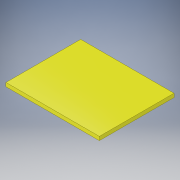
# Autodesk Inventor part: LargeCaseCaseTopForPiZeroWV02
Saved by Autodesk Inventor 2019.4 (Build 234330000, 330)
## iProperties
Created: 2018-12-18
Part Number: LargeCaseCaseTopForPiZeroWV02
Material: LCP Plastic
Document SubType Name: Modeling
Designer: steele
Density: 1.626 g/cm^3
Appearance: Yellow
PiZeroWLength: 2.559 in
PiZeroWWidth: 1.181 in
CaseLength: 3.150 in
CaseWidth: 1.772 in
CaseHeight: 0.515 in
PiZeroWMountingHole: 0.108 in
CaseWallThickness: 0.050 in
CaseFloorThickness: 0.200 in
PiZeroMoutingHolesLength: 2.283 in
PiZeroMountingHolesWidth: 0.906 in
PiZeroHoleSupport: 0.236 in
PiZeroWHoleHeight: 0.100 in
PiRibbonCableWidth: 0.787 in
PiRibbonCableThickness: 0.197 in
HdmiCenter: 0.748 in
MiniUsbCenter: 1.630 in
PowerCenter: 2.126 in
HdmiWidth: 1.102 in
MiniUsbWidth: 0.709 in
PowerWidth: 0.787 in
EndOfCaseToStartOfPiZero: 0.295 in
EyepieceOutsideDiameter: 1.250 in
EyepieceWallThickness: 0.075 in
EyepieceInnerDiameter: 1.100 in
PiRibbonCableHeightFromTp: 0.350 in
NutHeightPlusOffset: 0.073 in
NutWidthPlusOffset: 0.198 in
Author: steele
Autodesk Inventor part; units mm, degrees
ref_plane "YZ Plane" through (0, 0, 0) normal (1, 0, 0) x (0, 1, 0)
ref_plane "XZ Plane" through (0, 0, 0) normal (0, 1, 0) x (-1, 0, 0)
ref_plane "XY Plane" through (0, 0, 0) normal (0, 0, 1) x (1, 0, 0)
sketch "Sketch1" plane through (0, 0, 0) normal (0, 1, 0) x (-1, 0, 0)
  line L0 (63.5, 50.8) -> (-63.5, 50.8)
  line L1 (-63.5, 50.8) -> (-63.5, -50.8)
  line L2 (-63.5, -50.8) -> (63.5, -50.8)
  line L3 (63.5, -50.8) -> (63.5, 50.8)
  line L4 (63.5, 50.8) -> (-63.5, -50.8) construction
  line L5 (-63.5, 50.8) -> (63.5, -50.8) construction
  point P0 (0, 0)
  dimension "d0" = 127
  dimension "d1" = 101.6
  constraints: 12 end point, 2 midpoint, 2 parallel, 1 horizontal, 1 perpendicular
  measures "d0" distance of L1.end L2.end
  measures "d1" distance of L2.end L0.start
extrude "Extrusion1" add sketch "Sketch1" against normal blind 5.08
sketch "Sketch22" plane through (0, -5.08, 0) normal (0, -1, 0) x (1, 0, 0)
  point P0 (34.92, -17.42)
  point P1 (34.92, 17.42)
  point P2 (-34.92, 17.42)
  point P3 (-34.92, -17.42)
equation "\"d0\" = LargeCaseLength"
equation "\"d1\" = LargeCaseWidth"
equation "\"d2\" = CaseFloorThickness"
equation "\"PiZeroWLength\" = 65"
equation "\"PiZeroWWidth\" = 30"
equation "\"CaseLength\" = PiZeroWLength + 2 * EndOfCaseToStartOfPiZero"
equation "\"CaseWidth\" = PiZeroWWidth + 2 * EndOfCaseToStartOfPiZero"
equation "\"PiZeroWMountingHole\" = 2.75"
equation "\"CaseWallThickness\" = 1.27"
equation "\"CaseFloorThickness\" = 5.08"
equation "\"PiZeroMoutingHolesLength\" = 58"
equation "\"PiZeroMountingHolesWidth\" = 23"
equation "\"PiZeroHoleSupport\" = 6"
equation "\"PiZeroWHoleHeight\" = 2.54"
equation "\"PiRibbonCableWidth\" = 20"
equation "\"PiRibbonCableThickness\" = 5"
equation "\"HdmiCenter\" = 19"
equation "\"MiniUsbCenter\" = 41.4"
equation "\"PowerCenter\" = 54"
equation "\"HdmiWidth\" = 28"
equation "\"MiniUsbWidth\" = 18"
equation "\"PowerWidth\" = 20"
equation "\"EndOfCaseToStartOfPiZero\" = 7.5"
equation "\"EyepieceOutsideDiameter\" = 31.75"
equation "\"EyepieceWallThickness\" = 1.905"
equation "\"EyepieceInnerDiameter\" = EyepieceOutsideDiameter - 2 * EyepieceWallThickness"
equation "\"HeightOfConnectorHolesAboveBottom\" = 6"
equation "\"HdmiHightAboveBottom\" = 6"
equation "\"MiniUsbHeightAboveBottom\" = 5"
equation "\"PowerHeightAboveBottom\" = 5"
equation "\"PiRibbonCableHeightFromTp\" = 8.89"
equation "\"NutHeightPlusOffset\" = 1.8415"
equation "\"NutWidthPlusOffset\" = 5.0165"
equation "\"LargeCaseWidth\" = 101.6"
equation "\"LargeCaseLength\" = 127"
body "Solid1"
